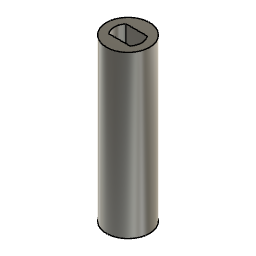
NEW extended Shaft 2 (Autodesk Fusion 360 design; units mm, degrees)
Autodesk Fusion 360 part; units mm, degrees
sketch "Sketch1" plane through (0, 0, 0) normal (0, 0, 1) x (1, 0, 0)
  circle A0 centre (0, 0) radius 4
  line L0 (0, 0) -> (0, 1.6)
  line L1 (0, 0) -> (0, -1.6)
  line L2 (-1.9879, 1.5971) -> (1.9879, 1.5971)
  line L3 (-1.9878, -1.5972) -> (1.9878, -1.5972)
  arc A1 (-1.9879, 1.5971) -> (-1.9878, -1.5972) centre (0, 0) ccw
  arc A2 (1.9878, -1.5972) -> (1.9879, 1.5971) centre (0, 0) ccw
  dimension "d1" = 8
  dimension "d2" = 5.1
  dimension "d3" = 1.6
  dimension "d4" = 1.6
  constraint coincident A0.centre L0.start
  constraint vertical L0
  constraint parallel L0 L1
  constraint perpendicular L0 L2
  constraint coincident L3.end A1
  constraint perpendicular L1 L3
  constraint concentric A1 A2
  measures "d1" diameter of A0
  measures "d2" diameter of A1
  measures "d3" distance of A0.centre L0.end
  measures "d4" distance of A0.centre L1.end
extrude "Extrude1" add sketch "Sketch1" along normal blind 30
